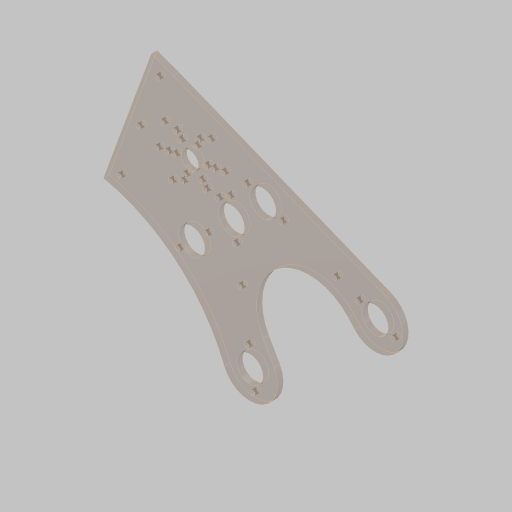
# Autodesk Inventor part: GP7-001
Saved by Autodesk Inventor 2023.5 (Build 275446000, 446)
## iProperties
Created: 2025-02-24
Part Number: GP7-001
Material: Polycarbonate, Smoke
Document SubType Name: Modeling
Designer: dlangdon
Density: 1.2 g/cm^3
Appearance: Polycarbonate - Smoked
Author: dlangdon
Autodesk Inventor part; units mm, degrees
ref_plane "YZ Plane" through (0, 0, 0) normal (1, 0, 0) x (0, 1, 0)
ref_plane "XZ Plane" through (0, 0, 0) normal (0, 1, 0) x (-1, 0, 0)
ref_plane "XY Plane" through (0, 0, 0) normal (0, 0, 1) x (1, 0, 0)
sketch "Sketch1" plane through (0, 0, 0) normal (0, 0, 1) x (1, 0, 0)
  circle A0 centre (68.1014, 57.1438) radius 38.1 construction
  circle A1 centre (-68.1014, -57.1438) radius 38.1 construction
  circle A2 centre (0, 0) radius 50.8 construction
  line L0 (-38.9151, -32.6536) -> (38.9151, 32.6536) construction
  line L1 (68.1014, 57.1438) -> (-68.1014, -57.1438) construction
  line L2 (-3.81, 6.5991) -> (-3.81, 50.6569) construction
  line L3 (-399.8199, -95.2438) -> (465.5721, -95.2438) construction
  circle A3 centre (151.5813, -38.0938) radius 57.15 construction
  circle A4 centre (68.1014, 57.1438) radius 14.2621
  circle A5 centre (-68.1014, -57.1438) radius 14.2621
  circle A6 centre (-3.81, 6.5991) radius 57.15 construction
  circle A7 centre (-68.1014, -57.1438) radius 30.1371 construction
  circle A8 centre (68.1014, 57.1438) radius 30.1371 construction
  circle A9 centre (-54.069, 106.0548) radius 14.2621
  line L4 (-54.069, 106.0548) -> (68.1014, 57.1438) construction
  circle A10 centre (68.1014, 57.1438) radius 14.2875 construction
  circle A11 centre (-68.1014, -57.1438) radius 14.2875 construction
  circle A12 centre (-88.3049, 72.8934) radius 14.2621
  line L5 (-68.1014, -57.1438) -> (-88.3049, 72.8934) construction
  circle A13 centre (-88.3049, 72.8934) radius 23.8316 construction
  circle A14 centre (-54.069, 106.0548) radius 23.8316 construction
  line L6 (38.7541, 44.736) -> (45.6559, 37.033)
  line L7 (-41.8356, -42.367) -> (-53.6186, -21.4227)
  arc A15 (38.7541, 44.736) -> (-53.6186, -21.4227) centre (-3.81, 6.5991) ccw
  line L8 (-175.4508, 186.3347) -> (-151.5826, 177.6474)
  line L9 (-151.5826, 177.6474) -> (-203.7064, 34.4382) construction
  line L10 (-203.7064, 34.4382) -> (-227.5746, 43.1256) construction
  line L11 (-227.5746, 43.1256) -> (-175.4508, 186.3347) construction
  line L12 (-254.1767, -29.9631) -> (29.2993, -133.1399) construction
  line L13 (-175.4508, 186.3347) -> (194.0315, 51.8542) construction
  line L14 (-175.4508, 186.3347) -> (-254.1767, -29.9631) construction
  circle A16 centre (-133.5197, 106.5946) radius 31.75 construction
  line L15 (-84.6462, 49.3444) -> (-73.9507, -19.4955) construction
  circle A17 centre (23.888, 74.8446) radius 9.525 construction
  line L16 (-163.5167, 181.9911) -> (-215.6405, 38.7819) construction
  line L17 (-168.9462, 167.0734) -> (-210.211, 53.6995) construction
  circle A18 centre (-133.5197, 106.5946) radius 17.4625 construction
  circle A19 centre (-133.5197, 106.5946) radius 9.525
  circle A20 centre (-54.069, 106.0548) radius 30.1816 construction
  line L18 (-175.4508, 186.3347) -> (-227.5746, 43.1256)
  arc A21 (45.6559, 37.033) -> (79.3119, 85.1182) centre (68.1014, 57.1438) ccw
  arc A22 (-96.1421, -68.1875) -> (-41.8356, -42.367) centre (-68.1014, -57.1438) ccw
  line L19 (-133.5197, 106.5946) -> (-116.3225, 109.627) construction
  line L20 (-97.5619, 112.935) -> (-169.4775, 100.2543) construction
  circle A23 centre (-169.4775, 100.2543) radius 4.7625 construction
  line L21 (0, 0) -> (-3.81, 6.5991) construction
  circle A24 centre (68.1014, 57.1438) radius 28.6512 construction
  line L22 (54.608, 31.8689) -> (-60.7858, 93.4733) construction
  line L23 (75.778, 84.7475) -> (-50.2477, 119.7954) construction
  line L24 (-151.5826, 177.6474) -> (79.3119, 85.1182)
  line L25 (-133.5197, 106.5946) -> (-131.3642, 31.5559) construction
  circle A25 centre (-131.3642, 31.5559) radius 31.75 construction
  circle A26 centre (-131.3642, 31.5559) radius 14.2621
  line L26 (-88.3049, 72.8934) -> (-131.3642, 31.5559) construction
  circle A27 centre (-133.5197, 106.5946) radius 25.4 construction
  arc A28 (-96.1421, -68.1875) -> (-227.5746, 43.1256) centre (-265.4783, -134.8799) ccw
  circle A29 centre (-133.5197, 106.5946) radius 36.5125 construction
  line L27 (-163.429, 127.5373) -> (-133.5197, 106.5946) construction
  point P0 (-79.2984, 14.9245)
  point P1 (-189.5786, 110.3865)
  point P2 (-189.5786, 110.3865)
  point P3 (-127.5472, 123.004)
  point P4 (-144.7444, 119.9717)
  point P5 (-150.7169, 103.5623)
  point P6 (-139.4922, 90.1853)
  point P7 (-122.295, 93.2176)
  point P8 (-108.5056, 111.0053)
  point P9 (-124.8324, 130.4628)
  point P10 (-149.8465, 126.0522)
  point P11 (-158.5338, 102.184)
  point P12 (-142.207, 82.7264)
  point P13 (-117.1929, 87.1371)
  point P14 (-139.86, 142.5524)
  point P15 (-169.4775, 100.2543)
  point P16 (-127.1794, 70.6368)
  point P17 (-112.577, 136.5039)
  point P18 (-154.4624, 76.6853)
  point P19 (-103.6104, 85.6519)
  dimension "d7" = 76.2
  dimension "d18" = 47.6631
  dimension "d34" = 34.925
  dimension "d65" = 50.8
  dimension "d3" = 50
  dimension "d4" = 0
  dimension "d8" = 101.6
  dimension "d9" = 28.5242
  dimension "d10" = 76.2
  dimension "d11" = 114.3
  dimension "d12" = 114.3
  dimension "d13" = 15.875
  dimension "d14" = 15.875
  dimension "d15" = 131.5974
  dimension "d16" = 28.575
  dimension "d17" = 131.5974
  dimension "d19" = 47.6631
  dimension "d22" = 25.4
  dimension "d23" = 152.4
  dimension "d26" = 230.1793
  dimension "d27" = 63.5
  dimension "d30" = 203.2
  dimension "d31" = 20
  dimension "d32" = 19.05
  dimension "d33" = 120.65
  dimension "d35" = 19.05
  dimension "d36" = 6.35
  dimension "d40" = 360
  dimension "d44" = 9.525
  dimension "d55" = 80
  dimension "d56" = 7.62
  dimension "d57" = 0
  dimension "d58" = 57.3024
  dimension "d59" = 63.5
  dimension "d60" = 75.0697
  dimension "d61" = 59.69
  dimension "d62" = 55
  dimension "d68" = 360
  dimension "d70" = 41.275
  dimension "d71" = 60
  dimension "d82" = 360
  dimension "d87" = 360
  dimension "d89" = 45
  constraints: 56 end point, 26 centre point, 24 coincident, 23 point on circle, 17 tangent, 7 midpoint, 5 collinear, 5 equal radius, 5 point on line, 3 parallel, 2 horizontal, 1 concentric, 1 perpendicular, 1 vertical, 39 other
  measures "d3" angle of L2 L0
  measures "d4" distance between parallel lines of L0 L1
  measures "d8" diameter of A2
  measures "d9" diameter of A4
  measures "d10" diameter of A0
  measures "d11" diameter of A3
  measures "d12" diameter of A6
  measures "d13" radial gap between concentric circles of A5 A7
  measures "d14" radial gap between concentric circles of A4 A8
  measures "d15" distance of L4.start L4.end
  measures "d16" diameter of A10
  measures "d17" distance of L5.start L5.end
  measures "d19" diameter of A14
  measures "d22" distance of L9.end L10.end
  measures "d23" distance of L10.end L8.start
  measures "d26" distance of L13.start L12.start
  measures "d27" diameter of A16
  measures "d30" distance from line of point (0, 0) L9
  measures "d31" angle of L3 L12
  measures "d32" diameter of A17
  measures "d33" distance of L17.start L17.end
  measures "d35" diameter of A19
  measures "d36" radial gap between concentric circles of A14 A20
  measures "d44" diameter of A23
  measures "d55" angle of L1 L21
  measures "d56" distance of L21.start L21.end
  measures "d57" distance between parallel lines of L13 L8
  measures "d58" diameter of A24
  measures "d59" diameter of A25
  measures "d60" distance of L19.start L25.end
  measures "d61" distance of L26.start L26.end
  measures "d62" angle of L15 L26
  measures "d70" distance from line of L9 L19.start
  measures "d71" angle of L9 L20
  measures "d89" angle of L20 L27
extrude "Extrusion1" add sketch "Sketch1" along normal blind 6.35
hole "Hole1" at (23.888, 74.8446, 0) at (-168.9462, 167.0734, 0) at (-189.5786, 110.3865, 0) at (-210.211, 53.6995, 0) at (-116.3225, 109.627, 0) at (-127.5472, 123.004, 0) at (-144.7444, 119.9717, 0) at (-150.7169, 103.5623, 0) at (-139.4922, 90.1853, 0) at (-122.295, 93.2176, 0) at (-97.5619, 112.935, 0) at (-169.4775, 100.2543, 0) at (-142.207, 82.7264, 0) at (-158.5338, 102.184, 0) at (-149.8465, 126.0522, 0) at (-124.8324, 130.4628, 0) at (-108.5056, 111.0053, 0) at (-117.1929, 87.1371, 0) at (-79.2984, 14.9245, 0) at (-163.429, 127.5373, 0) at (-112.577, 136.5039, 0) at (-103.6104, 85.6519, 0) at (-154.4624, 76.6853, 0) direction (0, 0, 1) diameter 5.1054 end through all clearance for "Flat Head Machine Screw (82)" size "#10" standard "Ansi Unified Screw Threads"
sketch "Sketch2" plane through (0, 0, 6.35) normal (0, 0, 1) x (1, 0, 0)
  circle A0 centre (-117.1929, 87.1371) radius 2.5527 construction
  circle A1 centre (-124.8324, 130.4628) radius 2.5527 construction
  circle A2 centre (-158.5338, 102.184) radius 2.5527 construction
  circle A3 centre (-169.4775, 100.2543) radius 2.5527 construction
  circle A4 centre (-122.295, 93.2176) radius 2.5527 construction
  circle A5 centre (-150.7169, 103.5623) radius 2.5527 construction
  circle A6 centre (-127.5472, 123.004) radius 2.5527 construction
  circle A7 centre (-210.211, 53.6995) radius 2.5527 construction
  circle A8 centre (-168.9462, 167.0734) radius 2.5527 construction
  circle A9 centre (23.888, 74.8446) radius 2.5527 construction
  circle A10 centre (-189.5786, 110.3865) radius 2.5527 construction
  circle A11 centre (-116.3225, 109.627) radius 2.5527 construction
  circle A12 centre (-144.7444, 119.9717) radius 2.5527 construction
  circle A13 centre (-139.4922, 90.1853) radius 2.5527 construction
  circle A14 centre (-97.5619, 112.935) radius 2.5527 construction
  circle A15 centre (-142.207, 82.7264) radius 2.5527 construction
  circle A16 centre (-149.8465, 126.0522) radius 2.5527 construction
  circle A17 centre (-108.5056, 111.0053) radius 2.5527 construction
  circle A18 centre (-79.2984, 14.9245) radius 2.5527 construction
  line L0 (-41.8356, -42.367) -> (-53.6186, -21.4227) construction
  arc A19 (38.7541, 44.736) -> (-53.6186, -21.4227) centre (-3.81, 6.5991) ccw construction
  line L1 (38.7541, 44.736) -> (45.6559, 37.033) construction
  arc A20 (45.6559, 37.033) -> (79.3119, 85.1182) centre (68.1014, 57.1438) ccw construction
  line L2 (79.3119, 85.1182) -> (-151.5826, 177.6474) construction
  line L3 (-151.5826, 177.6474) -> (-175.4508, 186.3347) construction
  line L4 (-175.4508, 186.3347) -> (-227.5746, 43.1256) construction
  arc A21 (-96.1421, -68.1875) -> (-227.5746, 43.1256) centre (-265.4783, -134.8799) ccw construction
  arc A22 (-96.1421, -68.1875) -> (-41.8356, -42.367) centre (-68.1014, -57.1438) ccw construction
  circle A23 centre (-88.3049, 72.8934) radius 14.2621 construction
  circle A24 centre (-133.5197, 106.5946) radius 9.525 construction
  circle A25 centre (-131.3642, 31.5559) radius 14.2621 construction
  circle A26 centre (-54.069, 106.0548) radius 14.2621 construction
  circle A27 centre (-68.1014, -57.1438) radius 14.2621 construction
  circle A28 centre (68.1014, 57.1438) radius 14.2621 construction
  line L5 (-71.3282, -36.3745) -> (-64.8745, -77.9131) construction
  line L6 (-146.5266, 16.9998) -> (-116.2019, 46.112) construction
  line L7 (-91.5318, 93.6628) -> (-85.0781, 52.1241) construction
  line L8 (-73.5818, 113.8667) -> (-34.5562, 98.2428) construction
  line L9 (48.5885, 64.9558) -> (87.6142, 49.3319) construction
  circle A29 centre (-88.3049, 72.8934) radius 14.2621 construction
  line L10 (-54.069, 106.0548) -> (-88.3049, 72.8934) construction
  line L11 (-54.069, 106.0548) -> (68.1014, 57.1438) construction
  line L12 (-88.3049, 72.8934) -> (-131.3642, 31.5559) construction
  line L13 (-88.3049, 72.8934) -> (-68.1014, -57.1438) construction
  circle A30 centre (-103.6104, 85.6519) radius 2.5527 projected
  point P0 (0, 0)
  point P1 (-116.0598, 70.5176)
  point P2 (-113.1961, 73.3575)
  dimension "d72" = 42.037
  constraints: 19 end point, 14 coincident, 5 collinear, 5 midpoint, 4 equal length, 1 other
  measures "d72" distance of L5.start L5.end
hole "Hole2" at (-71.3282, -36.3745, 6.35) at (-116.2019, 46.112, 6.35) at (-64.8745, -77.9131, 6.35) at (-146.5266, 16.9998, 6.35) at (-85.0781, 52.1241, 6.35) at (-91.5318, 93.6628, 6.35) at (-34.5562, 98.2428, 6.35) at (-73.5818, 113.8667, 6.35) at (87.6142, 49.3319, 6.35) at (48.5885, 64.9558, 6.35) direction (0, 0, -1) diameter 5.1054 end through all clearance for "Flat Head Machine Screw (82)" size "#10" standard "Ansi Unified Screw Threads"
body "Solid1"
